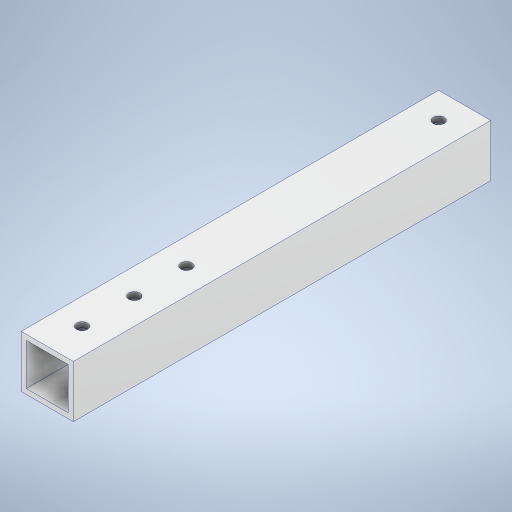
# Autodesk Inventor part: 射出_角柱1
Saved by Autodesk Inventor 2023 (Build 270158000, 158)
## iProperties
Created: 2022-04-19
Part Number: 射出_角柱1
Material: アルミニウム 6061
Document SubType Name: Modeling
Designer: yuta
Density: 2.7 g/cm^3
Appearance: アルミニウム - フラット
Author: yuta
Autodesk Inventor part; units mm, degrees
ref_plane "YZ Plane" through (0, 0, 0) normal (1, 0, 0) x (0, 1, 0)
ref_plane "XZ Plane" through (0, 0, 0) normal (0, 1, 0) x (-1, 0, 0)
ref_plane "XY Plane" through (0, 0, 0) normal (0, 0, 1) x (1, 0, 0)
sketch "スケッチ1" plane through (0, 0, 0) normal (0, 0, 1) x (1, 0, 0)
  line L0 (0, 0) -> (15, 0)
  line L1 (15, 0) -> (15, 15)
  line L2 (15, 15) -> (0, 15)
  line L3 (0, 15) -> (0, 0)
  dimension "d0" = 15
  dimension "d1" = 15
  constraints: 8 end point, 2 parallel, 1 horizontal, 1 perpendicular
  measures "d0" distance of L2.end L1.end
  measures "d1" distance of L1.end L0.end
extrude "押し出し1" add sketch "スケッチ1" along normal blind 50
sketch "スケッチ2" plane through (0, 15, 0) normal (0, 1, 0) x (1, 0, 0)
  circle A0 centre (7.5, -40) radius 1.6
  line L0 (15, 0) -> (15, -50) projected
  line L1 (15, -50) -> (0, -50) projected
  circle A1 centre (7.5, -25) radius 1.6
  circle A2 centre (7.5, -10) radius 1.6
  line L2 (15, 0) -> (0, 0) projected
  dimension "d4" = 3.2
  dimension "d5" = 7.5
  dimension "d6" = 10
  dimension "d7" = 3.2
  dimension "d8" = 3.2
  dimension "d9" = 15
  dimension "d10" = 7.5
  dimension "d11" = 15
  dimension "d12" = 10
  dimension "d13" = 7.5
  constraints: 3 centre point
  measures "d4" diameter of A0
  measures "d5" distance from line of L0 A0.centre
  measures "d6" distance from line of L1 A0.centre
  measures "d7" diameter of A1
  measures "d8" diameter of A2
  measures "d9" distance of A1.centre A0.centre
  measures "d10" distance from line of L0 A1.centre
  measures "d11" distance of A1.centre A2.centre
  measures "d12" distance from line of L2 A2.centre
  measures "d13" distance from line of L0 A2.centre
hole "穴1" at (7.5, 15, 40) at (7.5, 15, 25) at (7.5, 15, 10) direction (0, -1, 0) diameter 3.2 end through all
sketch "スケッチ3" plane through (0, 0, 0) normal (0, 0, -1) x (-1, 0, 0)
  line L0 (0, 15) -> (0, 0) projected
  line L1 (0, 0) -> (-15, 0)
  line L2 (-15, 0) -> (-15, 15)
  line L3 (-15, 15) -> (0, 15)
  line L4 (0, 15) -> (0, 0)
  dimension "d21" = 15
  dimension "d22" = 15
  constraints: 8 end point, 2 parallel, 1 horizontal, 1 perpendicular
  measures "d21" distance of L2.end L3.end
  measures "d22" distance of L1.end L2.end
extrude "押し出し2" add sketch "スケッチ3" along normal blind 135
sketch "スケッチ4" plane through (0, 15, 50) normal (0, 1, 0) x (1, 0, 0)
  line L0 (15, 0) -> (15, 185) projected
  line L1 (15, 185) -> (0, 185)
  line L2 (0, 185) -> (0, 105)
  line L3 (0, 105) -> (15, 105)
  line L4 (15, 105) -> (15, 185)
  point P0 (0, 50)
  dimension "d25" = 15
  dimension "d26" = 80
  constraints: 8 end point, 2 parallel, 1 horizontal, 1 perpendicular
  measures "d25" distance of L3.end L2.end
  measures "d26" distance of L2.end L1.end
extrude "押し出し3" cut sketch "スケッチ4" against normal blind 135
sketch "スケッチ5" plane through (15, 15, -55) normal (0, 0, -1) x (-1, 0, 0)
  line L0 (15, 0) -> (15, -15) projected
  line L1 (0, -15) -> (0, 0) projected
  line L2 (15, -15) -> (0, -15)
  line L3 (0, -15) -> (0, 0)
  line L4 (0, 0) -> (15, 0)
  line L5 (15, 0) -> (15, -15)
  constraints: 8 end point, 2 parallel, 1 horizontal, 1 perpendicular
extrude "押し出し4" add sketch "スケッチ5" along normal blind 15
sketch "スケッチ6" plane through (0, 15, 50) normal (0, 1, 0) x (1, 0, 0)
  line L0 (15, 120) -> (15, 0) construction
  line L1 (15, 120) -> (0, 120) construction
  line L2 (0, 120) -> (0, 105) construction
  line L3 (0, 105) -> (15, 105) construction
  line L4 (15, 105) -> (15, 120) construction
  circle A0 centre (7.5, 112.5) radius 1.6
  point P0 (0, 50)
  dimension "d31" = 15
  dimension "d32" = 15
  dimension "d33" = 3.2
  constraints: 8 end point, 2 parallel, 1 centre point, 1 horizontal, 1 perpendicular
  measures "d31" distance of L3.end L2.end
  measures "d32" distance of L2.end L1.end
  measures "d33" diameter of A0
hole "穴2" at (7.5, 15, -62.5) direction (0, -1, 0) diameter 3.2 end through all
sketch "スケッチ7" plane through (0, 0, 50) normal (0, 0, 1) x (1, 0, 0)
  line L0 (1.5, 1.5) -> (13.5, 1.5)
  line L1 (13.5, 1.5) -> (13.5, 13.5)
  line L2 (13.5, 13.5) -> (1.5, 13.5)
  line L3 (1.5, 13.5) -> (1.5, 1.5)
  line L4 (15, 15) -> (0, 15) projected
  line L5 (0, 15) -> (0, 0) projected
  point P0 (0, 7.5)
  point P1 (1.5, 7.5)
  dimension "d41" = 12
  dimension "d42" = 12
  dimension "d43" = 1.5
  dimension "d44" = 1.5
  constraints: 8 end point, 2 midpoint, 2 parallel, 1 horizontal, 1 perpendicular
  measures "d41" distance of L2.end L1.end
  measures "d42" distance of L1.end L0.end
  measures "d43" distance between parallel lines of L4 L2
  measures "d44" distance of point (0, 7.5) point (1.5, 7.5)
extrude "押し出し5" cut sketch "スケッチ7" against normal blind 130
